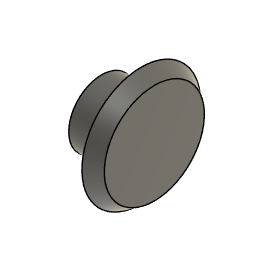
Rivet_ (Autodesk Fusion 360 design; units mm, degrees)
Autodesk Fusion 360 part; units mm, degrees
sketch "Sketch1" plane through (0, 0, 0) normal (0, 1, 0) x (1, 0, 0)
  line L0 (0, 0) -> (101.6, 0)
  line L1 (101.6, 0) -> (101.6, -96.5147)
  line L2 (101.6, -96.5147) -> (76.2, -114.3)
  line L3 (76.2, -114.3) -> (76.2, -63.5)
  line L4 (76.2, -63.5) -> (0, -63.5)
  line L5 (0, -63.5) -> (0, 0)
  dimension "d1" = 101.6
  dimension "d2" = 76.2
  dimension "d3" = 55
  dimension "d4" = 127
  dimension "d5" = 228.6
  constraint coincident L0.start L5.end
  constraint horizontal L0
  constraint perpendicular L0 L3
  constraint perpendicular L3 L4
  constraint vertical L1
  constraint vertical L5
  measures "d1" distance of L0.start L0.end
  measures "d2" distance of L3.end L4.end
  measures "d3" angle of L2 L3
revolve "Revolve1" add sketch "Sketch1" angle 360 about axis through (0, 0, 0) along (1, 0, 0)
